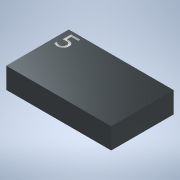
# Autodesk Inventor part: 5gram weight
Saved by Autodesk Inventor 2022 (Build 260153000, 153)
## iProperties
Created: 2021-08-25
Part Number: 5gram weight
Material: Generic
Document SubType Name: Modeling
Designer: benka
Density: 1 g/cm^3
Appearance: Default
Author: benka
Autodesk Inventor part; units mm, degrees
ref_plane "YZ Plane" through (0, 0, 0) normal (1, 0, 0) x (0, 1, 0)
ref_plane "XZ Plane" through (0, 0, 0) normal (0, 1, 0) x (-1, 0, 0)
ref_plane "XY Plane" through (0, 0, 0) normal (0, 0, 1) x (1, 0, 0)
sketch "Sketch1" plane through (0, 0, 0) normal (0, 1, 0) x (-1, 0, 0)
  line L0 (9.525, -5.675) -> (-9.525, -5.675)
  line L1 (-9.525, -5.675) -> (-9.525, 5.675)
  line L2 (-9.525, 5.675) -> (9.525, 5.675)
  line L3 (9.525, 5.675) -> (9.525, -5.675)
  point P0 (0, 0)
  point P1 (0, 0)
  dimension "d0" = 19.05
  dimension "d1" = 11.35
  constraints: 8 end point, 2 parallel, 1 horizontal, 1 perpendicular
  measures "d0" distance of L1.end L2.end
  measures "d1" distance of L0.end L1.end
extrude "Extrusion1" add sketch "Sketch1" along normal blind 3.8
sketch "Sketch2" plane through (0, 3.8, 0) normal (0, 1, 0) x (1, 0, 0)
  line L0 (-8.9301, 5.134) -> (-6.6428, 5.134) construction
  line L1 (-6.6428, 5.134) -> (-6.6428, 2.0218) construction
  line L2 (-6.6428, 2.0218) -> (-8.9301, 2.0218) construction
  line L3 (-8.9301, 2.0218) -> (-8.9301, 5.134) construction
  spline S0 degree 2 poles (-6.8602, 3.0543) (-6.8602, 2.8344) (-7.001, 2.459) (-7.1294, 2.3207) knots 0 0 0 1 2 2 2
  spline S1 degree 2 poles (-7.1294, 2.3207) (-7.2579, 2.1823) (-7.6407, 2.0218) (-7.8778, 2.0218) knots 0 0 0 1 2 2 2
  spline S2 degree 2 poles (-7.8778, 2.0218) (-8.0952, 2.0218) (-8.52, 2.1181) (-8.6757, 2.1947) knots 0 0 0 1 2 2 2
  line L4 (-8.6757, 2.1947) -> (-8.6757, 2.6269)
  line L5 (-8.6757, 2.6269) -> (-8.646, 2.6269)
  spline S3 degree 2 poles (-8.646, 2.6269) (-8.5991, 2.5924) (-8.4237, 2.5034) (-8.3175, 2.4639) knots 0 0 0 1 2 2 2
  spline S4 degree 2 poles (-8.3175, 2.4639) (-8.1965, 2.4219) (-7.9964, 2.375) (-7.8704, 2.375) knots 0 0 0 1 2 2 2
  spline S5 degree 2 poles (-7.8704, 2.375) (-7.7469, 2.375) (-7.5147, 2.4639) (-7.4308, 2.5603) knots 0 0 0 1 2 2 2
  spline S6 degree 2 poles (-7.4308, 2.5603) (-7.3542, 2.6516) (-7.2752, 2.8937) (-7.2752, 3.0567) knots 0 0 0 1 2 2 2
  spline S7 degree 2 poles (-7.2752, 3.0567) (-7.2752, 3.2197) (-7.3641, 3.4272) (-7.4481, 3.4964) knots 0 0 0 1 2 2 2
  spline S8 degree 2 poles (-7.4481, 3.4964) (-7.5345, 3.573) (-7.7914, 3.6372) (-7.947, 3.6372) knots 0 0 0 1 2 2 2
  spline S9 degree 2 poles (-7.947, 3.6372) (-8.115, 3.6372) (-8.4484, 3.5853) (-8.5497, 3.5631) knots 0 0 0 1 2 2 2
  line L6 (-8.5497, 3.5631) -> (-8.5497, 5.134)
  line L7 (-8.5497, 5.134) -> (-6.8775, 5.134)
  line L8 (-6.8775, 5.134) -> (-6.8775, 4.7759)
  line L9 (-6.8775, 4.7759) -> (-8.157, 4.7759)
  line L10 (-8.157, 4.7759) -> (-8.157, 3.9632)
  spline S10 degree 2 poles (-8.157, 3.9632) (-8.0829, 3.9731) (-7.9396, 3.9805) (-7.8803, 3.9805) knots 0 0 0 1 2 2 2
  spline S11 degree 2 poles (-7.8803, 3.9805) (-7.6457, 3.9805) (-7.3221, 3.9039) (-7.1739, 3.7903) knots 0 0 0 1 2 2 2
  spline S12 degree 2 poles (-7.1739, 3.7903) (-7.0232, 3.6767) (-6.8602, 3.3309) (-6.8602, 3.0543) knots 0 0 0 1 2 2 2
  point P0 (0, 0)
  constraints: 2 other
emboss "Emboss1" sketch "Sketch2" operation cut depth 0.3 direction (0, -1, 0)
body "Solid1"
